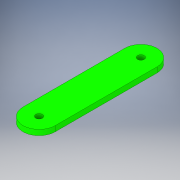
# Autodesk Inventor part: Outer Arm
Saved by Autodesk Inventor 2017 (Build 210142000, 142)
## iProperties
Created: 2017-03-25
Part Number: Outer Arm
Material: Generic
Document SubType Name: Modeling
Designer: Parshant Bombhi
Density: 1 g/cm^3
Appearance: Default(2)
Outer_Arm_Length: 6.250 in
Outer_Arm_Thickness: 0.250 in
Author: Parshant Bombhi
Autodesk Inventor part; units mm, degrees
ref_plane "YZ Plane" through (0, 0, 0) normal (1, 0, 0) x (0, 1, 0)
ref_plane "XZ Plane" through (0, 0, 0) normal (0, 1, 0) x (-1, 0, 0)
ref_plane "XY Plane" through (0, 0, 0) normal (0, 0, 1) x (1, 0, 0)
sketch "Sketch1" plane through (0, 0, 0) normal (0, 1, 0) x (-1, 0, 0)
  line L0 (0, -19.05) -> (0, -139.7)
  line L1 (19.05, -158.75) -> (19.05, -158.75)
  line L2 (38.1, -139.7) -> (38.1, -19.05)
  line L3 (19.05, 0) -> (19.05, 0)
  arc A0 (0, -139.7) -> (19.05, -158.75) centre (19.05, -139.7) ccw
  arc A1 (19.05, -158.75) -> (38.1, -139.7) centre (19.05, -139.7) ccw
  arc A2 (38.1, -19.05) -> (19.05, 0) centre (19.05, -19.05) ccw
  arc A3 (19.05, 0) -> (0, -19.05) centre (19.05, -19.05) ccw
  circle A4 centre (19.05, -19.05) radius 3.9688
  circle A5 centre (19.05, -139.7) radius 3.9688
  point P0 (0, 0)
  point P1 (0, -158.75)
  point P2 (38.1, -158.75)
  dimension "d0" = 38.1
  dimension "Outer_Arm_Length" = 158.75
  dimension "d2" = 19.05
  dimension "Shaft_Diameter" = 7.9375
  dimension "Pencil_Diameter" = 7.9375
  constraints: 8 end point, 8 point on circle, 8 tangent, 6 centre point, 6 point on line, 3 equal radius, 3 perpendicular, 2 coincident, 1 vertical
  measures "d0" distance of point (0, -158.75) point (38.1, -158.75)
  measures "Outer_Arm_Length" distance of point (0, 0) point (0, -158.75)
  measures "d2" radius of A0
  measures "Shaft_Diameter" diameter of A4
  measures "Pencil_Diameter" diameter of A5
extrude "Extrusion1" add sketch "Sketch1" along normal blind 6.35
body "Solid1"
